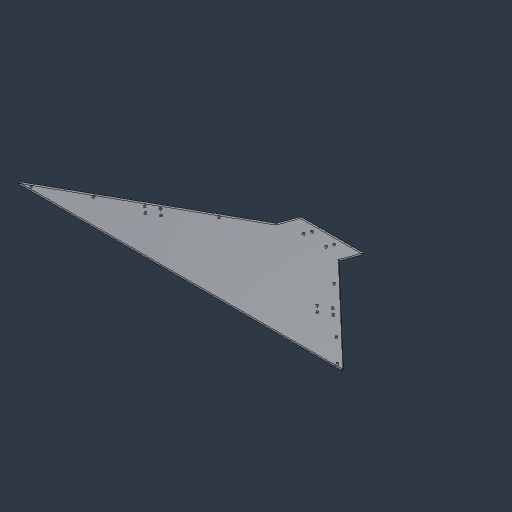
# Autodesk Inventor part: hopper_back
Saved by Autodesk Inventor 2024.3 (Build 283343000, 343)
## iProperties
Created: 2025-03-07
Part Number: hopper_back
Material: Polycarbonate, Clear
Document SubType Name: Sheet Metal
Designer: marcu
Density: 1.2 g/cm^3
Sheet Metal Rule: Default
Appearance: Polycarbonate - Clear
Author: marcu
Autodesk Inventor part; units mm, degrees
ref_plane "YZ Plane" through (0, 0, 0) normal (1, 0, 0) x (0, 1, 0)
ref_plane "XZ Plane" through (0, 0, 0) normal (0, 1, 0) x (-1, 0, 0)
ref_plane "XY Plane" through (0, 0, 0) normal (0, 0, 1) x (1, 0, 0)
ref_plane "Work Plane1" through (-1041.8338, 286.0261, 217.3698) normal (0, 0.9659258, -0.258819) x (0.7071068, -0.1830127, -0.6830127)
sketch "Sketch1" plane through (-1041.8338, 286.0261, 217.3698) normal (0, 0.9659258, -0.258819) x (0.7071068, -0.1830127, -0.6830127)
  line L0 (110.8111, -517.2111) -> (110.8111, -110.8111) construction
  line L1 (109.9183, -108.6558) -> (2.1553, -0.8927) construction
  line L2 (107.7631, -517.2111) -> (-203.2, -206.248) construction
  line L3 (2.1553, -0.8927) -> (110.8111, -109.5486)
  line L4 (110.8111, -109.5486) -> (110.8111, -517.2111)
  line L5 (110.8111, -517.2111) -> (107.7631, -517.2111)
  line L6 (107.7631, -517.2111) -> (-203.2, -206.248)
  line L7 (56.4832, -55.2206) -> (-148.8721, -260.5759) construction
  line L8 (110.8111, -109.5486) -> (2.1553, -0.8927)
  line L9 (2.1553, -0.8927) -> (-405.5073, -0.8927)
  line L10 (-405.5073, -0.8927) -> (-405.5073, -3.9407)
  line L11 (-405.5073, -3.9407) -> (-94.5442, -314.9038)
  line L12 (110.8111, -109.5486) -> (155.7124, -64.6473)
  line L13 (155.7124, -64.6473) -> (47.0565, 44.0085)
  line L14 (47.0565, 44.0085) -> (2.1553, -0.8927)
  line L15 (2.1553, -0.8927) -> (110.8111, -109.5486)
  point P0 (937.5005, -535.875)
  point P1 (2.1553, -0.8927)
  point P2 (-203.2, -206.248)
  point P3 (110.8111, -109.5486)
  dimension "d1" = 63.5
  measures "d1" distance of L8.start L12.end
extrude "Plate1" add sketch "Sketch1" along normal blind 3.048
sketch "Sketch2" plane through (-1041.8338, 288.9702, 216.5809) normal (0, 0.9659258, -0.258819) x (0.7071068, 0.1830127, 0.6830127)
  line L0 (-44.0085, 47.0565) -> (64.6473, 155.7124) construction
  line L1 (64.6473, 155.7124) -> (109.5486, 110.8111) construction
  line L2 (10.3194, 101.3844) -> (24.957, 86.7468) construction
  point P0 (535.875, 937.5005)
  point P1 (42.8728, 104.752)
  point P2 (6.9518, 68.831)
  point P3 (56.3432, 91.2817)
  point P4 (20.4222, 55.3606)
  dimension "d2" = 20.6375
  dimension "d3" = 20.6375
  dimension "d4" = 50.8
  dimension "d7" = 19.05
  dimension "d12" = 25.4
  constraints: 2 end point, 1 midpoint, 1 perpendicular, 3 other
  measures "d2" distance from line of point (42.873, 104.752) L0
  measures "d3" distance from line of L0 point (6.952, 68.831)
  measures "d4" distance of point (6.952, 68.831) point (42.873, 104.752)
  measures "d7" distance of point (42.873, 104.752) point (56.343, 91.282)
  measures "d12" distance from line of L2 point (42.873, 104.752)
hole "Hole1" at (-937.4473, 277.6455, 174.3166) at (-988.2473, 277.6455, 174.3166) at (-937.4473, 282.576, 192.7175) at (-988.2473, 282.576, 192.7175) direction (0, -0.9659258, 0.258819) diameter 5.1054 end through all clearance for "Flat Head Machine Screw (82)" size "#10" standard "Ansi Unified Screw Threads"
sketch "Sketch3" plane through (-1041.8338, 288.9702, 216.5809) normal (0, 0.9659258, -0.258819) x (0.7071068, 0.1830127, 0.6830127)
  circle A0 centre (56.3432, 91.2817) radius 2.5527 construction
  circle A1 centre (42.8728, 104.752) radius 2.5527 construction
  circle A2 centre (6.9518, 68.831) radius 2.5527 construction
  circle A3 centre (20.4222, 55.3606) radius 2.5527 construction
  line L0 (517.2111, 110.8111) -> (517.2111, 107.7631) construction
  line L1 (109.5486, 110.8111) -> (517.2111, 110.8111) construction
  line L2 (64.6473, 155.7124) -> (109.5486, 110.8111) construction
  line L3 (-44.0085, 47.0565) -> (64.6473, 155.7124) construction
  line L4 (0.8927, 2.1553) -> (-44.0085, 47.0565) construction
  line L5 (0.8927, -405.5073) -> (0.8927, 2.1553) construction
  line L6 (3.9407, -405.5073) -> (0.8927, -405.5073) construction
  line L7 (517.2111, 107.7631) -> (3.9407, -405.5073) construction
  line L8 (10.3194, 101.3844) -> (260.5759, -148.8721) construction
  line L9 (313.3798, 110.8111) -> (313.3798, 98.1111) construction
  line L10 (109.5486, 110.8111) -> (517.2111, 110.8111) construction
  point P0 (535.875, 937.5005)
  point P1 (287.9798, 98.1111)
  point P2 (313.3798, 72.7111)
  point P3 (287.9798, 72.7111)
  point P4 (13.5927, -201.676)
  point P5 (13.5927, -176.276)
  point P6 (38.9927, -201.676)
  point P7 (38.9927, -176.276)
  dimension "d20" = 12.7
  dimension "d23" = 25.4
  dimension "d26" = 25.4
  constraints: 4 end point, 4 symmetric about line, 3 midpoint, 2 perpendicular, 1 coincident, 1 horizontal, 1 vertical, 3 other
  measures "d20" distance of L9.start L9.end
  measures "d23" distance of point (313.38, 98.111) point (287.98, 98.111)
  measures "d26" distance of point (313.38, 98.111) point (313.38, 72.711)
hole "Hole2" at (-750.8658, 328.3671, 363.6122) at (-768.8263, 323.7186, 346.2637) at (-768.8263, 333.0157, 380.9607) at (-786.7868, 328.3671, 363.6122) at (-1156.8682, 333.0157, 380.9607) at (-1138.9077, 328.3671, 363.6122) at (-1174.8287, 328.3671, 363.6122) at (-1156.8682, 323.7186, 346.2637) direction (0, -0.9659258, 0.258819) diameter 5.1054 end through all clearance for "Flat Head Machine Screw (82)" size "#10" standard "Ansi Unified Screw Threads"
sketch "Sketch4" plane through (-1041.8338, 288.9702, 216.5809) normal (0, 0.9659258, -0.258819) x (0.7071068, 0.1830127, 0.6830127)
  line L0 (109.5486, 110.8111) -> (64.6473, 155.7124) projected
  line L1 (109.5486, 110.8111) -> (100.5683, 110.8111)
  line L2 (109.5486, 110.8111) -> (517.2111, 110.8111) projected
  line L3 (100.5683, 110.8111) -> (60.1571, 151.2222)
  line L4 (-44.0085, 47.0565) -> (64.6473, 155.7124) projected
  line L5 (64.6473, 155.7124) -> (60.1571, 151.2222)
  point P0 (535.875, 937.5005)
  dimension "d36" = 6.35
  constraints: 6 end point, 1 collinear, 1 perpendicular, 1 point on line
  measures "d36" distance between parallel lines of L0 L3
extrude "Cut1" cut sketch "Sketch4" against normal blind 3.048
ref_plane "Work Plane2" through (-962.8473, 265.9096, 142.2942) normal (1, 0, 0) x (0, -0.9659258, 0.258819)
mirror "Mirror1" about plane through (-962.8473, 265.9096, 142.2942) normal (1, 0, 0) of "Cut1"
sketch "Sketch5" plane through (-1041.8338, 288.9702, 216.5809) normal (0, 0.9659258, -0.258819) x (0.7071068, 0.1830127, 0.6830127)
  line L0 (100.5683, 110.8111) -> (517.2111, 110.8111) projected
  line L1 (517.2111, 101.9084) -> (109.471, 101.9084) construction
  line L2 (517.2111, 110.8111) -> (517.2111, 107.7631) projected
  line L3 (100.5683, 110.8111) -> (60.1571, 151.2222) projected
  point P0 (535.875, 937.5005)
  point P1 (498.1611, 101.9084)
  point P2 (396.5611, 101.9084)
  point P3 (193.3611, 101.9084)
  dimension "d40" = 8.9027
  dimension "d41" = 101.6
  dimension "d42" = 19.05
  dimension "d45" = 203.2
  constraints: 5 point on line, 2 end point, 1 parallel
  measures "d40" distance between parallel lines of L0 L1
  measures "d41" distance of point (498.161, 101.908) point (396.561, 101.908)
  measures "d42" distance of L1.start point (498.161, 101.908)
  measures "d45" distance of point (396.561, 101.908) point (193.361, 101.908)
hole "Hole3" at (-617.5206, 361.4895, 487.2266) at (-689.3626, 342.8954, 417.8325) at (-833.0467, 305.7072, 279.0443) direction (0, -0.9659258, 0.258819) diameter 5.1054 end through all
mirror "Mirror2" about plane through (-962.8473, 265.9096, 142.2942) normal (1, 0, 0) of "Hole3"
equation "\"d3\" = d2"
equation "\"d18\" = Thickness"
equation "\"d37\" = Thickness"
equation "\"d51\" = Thickness"
equation "\"d0\" = Thickness"
equation "\"BendRadius\" = Thickness"
equation "\"BendReliefWidth\" = Thickness"
equation "\"BendReliefDepth\" = 0.5 * Thickness"
equation "\"CornerReliefSize\" = 4 * Thickness"
equation "\"MinimumRemnant\" = 2 * Thickness"
equation "\"TransitionRadius\" = BendRadius"
equation "\"JacobiRadiusSize\" = BendRadius"
equation "\"GapSize\" = Thickness"
equation "\"Thickness\" = 3.048"
body "Solid1"
